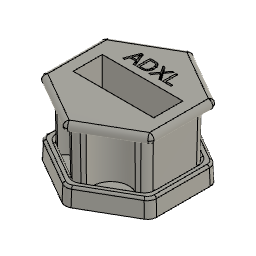
EXPAND CONNECTER v5 (Autodesk Fusion 360 design; units mm, degrees)
Autodesk Fusion 360 part; units mm, degrees
sketch "草图1" plane through (0, 0, 0) normal (0, 0, 1) x (1, 0, 0)
  line L0 (10.3777, -5.9969) -> (10.3823, 5.9889)
  line L1 (10.3823, 5.9889) -> (0.0046, 11.9858)
  line L2 (0.0046, 11.9858) -> (-10.3777, 5.9969)
  line L3 (-10.3777, 5.9969) -> (-10.3823, -5.9889)
  line L4 (-10.3823, -5.9889) -> (-0.0046, -11.9858)
  line L5 (-0.0046, -11.9858) -> (10.3777, -5.9969)
  line L6 (9, -3.25) -> (-9, -3.25)
  line L7 (-9, -3.25) -> (-9, 3.25)
  line L8 (-9, 3.25) -> (9, 3.25)
  line L9 (9, 3.25) -> (9, -3.25)
  line L10 (9, -3.25) -> (-9, 3.25) construction
  line L11 (-9, -3.25) -> (9, 3.25) construction
  line L12 (8, 2.925) -> (-8, 2.925) construction
  line L13 (-8, 3.25) -> (-8, -2.925) construction
  line L14 (-8, -2.925) -> (8, -2.925) construction
  line L15 (8, -2.925) -> (8, 3.25) construction
  line L16 (8, 2.925) -> (-8, -2.925) construction
  line L17 (-8, 2.925) -> (8, -2.925) construction
  line L18 (8, 3.25) -> (-8, 3.25)
  line L19 (-8, 3.25) -> (-8, -2.6)
  line L20 (-8, -2.6) -> (8, -2.6)
  line L21 (8, -2.6) -> (8, 3.25)
  line L22 (-12.3772, 7.1524) -> (-12.3828, -7.1428)
  line L23 (-12.3828, -7.1428) -> (-0.0055, -14.2952)
  line L24 (-0.0055, -14.2952) -> (12.3772, -7.1524)
  line L25 (12.3772, -7.1524) -> (12.3828, 7.1428)
  line L26 (12.3828, 7.1428) -> (0.0055, 14.2952)
  line L27 (0.0055, 14.2952) -> (-12.3772, 7.1524)
  circle A0 centre (-5.1935, -8.9873) radius 4
  circle A1 centre (5.1865, -8.9914) radius 4
  circle A2 centre (-5.1865, 8.9914) radius 4
  circle A3 centre (5.1935, 8.9873) radius 4
  line L28 (-5.1935, -8.9873) -> (-1.8781, -3.25) construction
  line L29 (5.1865, -8.9914) -> (1.8747, -3.25) construction
  point P0 (-3.5358, -6.1187)
  point P1 (3.5306, -6.1207)
  dimension "d5" = 10.38
  dimension "d6" = 18
  dimension "d7" = 6.5
  dimension "d8" = 16
  dimension "d9" = 5.85
  dimension "d10" = 5.85
  dimension "d11" = 2
  dimension "d28" = 8
  dimension "d29" = 8
  dimension "d30" = 8
  dimension "d31" = 8
  constraint horizontal L6
  constraint perpendicular L6 L7
  constraint parallel L6 L8
  constraint parallel L7 L9
  constraint coincident L10 origin
  constraint coincident L11 origin
  constraint horizontal L12
  constraint perpendicular L12 L13
  constraint parallel L12 L14
  constraint parallel L13 L15
  constraint coincident L16 origin
  constraint coincident L17 origin
  constraint coincident L12.end L13
  constraint coincident L8 L13.start
  constraint coincident L12.start L15
  constraint coincident L8 L15.end
  constraint horizontal L18
  constraint vertical L19
  constraint horizontal L20
  constraint vertical L21
  constraint midpoint L4 A0.centre
  constraint midpoint L5 A1.centre
  constraint midpoint L2 A2.centre
  constraint midpoint L1 A3.centre
  constraint coincident A0.centre L28.start
  constraint coincident L6 L28.end
  constraint perpendicular L4 L28
  constraint coincident A1.centre L29.start
  constraint coincident L6 L29.end
  constraint perpendicular L5 L29
  constraint midpoint L28 P0
  constraint midpoint L29 P1
  measures "d5" distance of origin L5
  measures "d6" distance of L7.end L8.end
  measures "d7" distance of L6.end L7.end
  measures "d8" distance of L13.end L14.end
  measures "d9" distance of L12.end L13.end
  measures "d10" distance of L15.end L20.end
  measures "d28" diameter of A0
  measures "d29" diameter of A1
  measures "d30" diameter of A2
  measures "d31" diameter of A3
extrude "拉伸1" add sketch "草图1" along normal blind 14.2 draft 1 contours L0 L1 L2 L3 L4 L5 A0 A1 A2 A3 | L5 A1 | L1 A3 | L4 A0 | L2 A2 | L6 L7 L8 L9 L19 L20 L21 | L8 L18 L19 L20 L21 makes body 1
extrude "拉伸2" add sketch "草图1" along normal blind 2 from surface at 14.2 contours L0 L1 L2 L3 L4 L5 A0 A1 A2 A3 | L0 L1 L5 L24 L25 L26 A1 A3 | L5 L24 A1 | L5 A1 | L1 A3 | L1 L26 A3 | L4 L5 L23 L24 A0 A1 | L1 L2 L26 L27 A2 A3 | L4 L23 A0 | L4 A0 | L2 A2 | L2 L27 A2 | L2 L3 L4 L22 L23 L27 A0 A2 bodies 1
extrude "拉伸3" cut sketch "草图1" along normal blind 7.8 contours L8 L18 L19 L20 L21 bodies 1
extrude "拉伸4" cut sketch "草图1" along normal blind 12 from surface at 7.8 contours L6 L7 L8 L9 L19 L20 L21 | L8 L18 L19 L20 L21 bodies 1
fillet "圆角1" radius 2 1 edges at (-0.0047, -12.1289, 7.1) on bodies 1
fillet "圆角2" radius 2 5 edges at (10.5063, 6.0604, 7.1) (10.5016, -6.0685, 7.1) (0.0047, 12.1289, 7.1) (-10.5016, 6.0685, 7.1) (-10.5063, -6.0604, 7.1) on bodies 1
fillet "圆角3" radius 1 18 edges at (-0.0055, -14.2952, 15.2) (12.3772, -7.1524, 15.2) (12.3828, 7.1428, 15.2) (0.0055, 14.2952, 15.2) (-12.3772, 7.1524, 15.2) (-12.3828, -7.1428, 15.2) (-6.1941, -10.719, 16.2) (-6.1941, -10.719, 14.2) (6.1859, -10.7238, 14.2) (6.1859, -10.7238, 16.2) (-12.38, 0.0048, 14.2) (-12.38, 0.0048, 16.2) (12.38, -0.0048, 16.2) (12.38, -0.0048, 14.2) (6.1941, 10.719, 16.2) (6.1941, 10.719, 14.2) (-6.1859, 10.7238, 16.2) (-6.1859, 10.7238, 14.2) on bodies 1
extrude "拉伸5" cut sketch "草图1" along normal blind 12 from surface at 2 contours L5 L24 A1 | L5 A1 | L1 A3 | L1 L26 A3 | L4 L23 A0 | L4 A0 | L2 A2 | L2 L27 A2 bodies 1
sketch "草图2" plane through (0, 0, 0) normal (0, 0, 1) x (1, 0, 0)
  line L0 (-6.0005, 4.5625) -> (7.0007, 4.5463) construction
  line L1 (7.0007, 4.5463) -> (7.0048, 7.8088) construction
  line L2 (7.0048, 7.8088) -> (-5.9964, 7.8251) construction
  line L3 (-5.9964, 7.8251) -> (-6.0005, 4.5625) construction
  point P0 (-5.9964, 7.8251)
  dimension "d40" = 3
  text T0 "ADXL" font "Arial" height 3 align left top in box 13.0012 x 3.2625 at (-6.0005, 4.5625) x (0.999999, -0.001251) y (0.001251, 0.999999) spacing 1
  constraint coincident P0
extrude "拉伸7" cut sketch "草图2" against normal blind 1 from surface at 16.2 text T0 bodies 1
sketch "草图3" plane through (0, 0, 0) normal (0, 0, 1) x (1, 0, 0)
  line L0 (-5.9964, 4.5463) -> (7.0007, 4.5463) construction
  line L1 (7.0007, 4.5463) -> (7.0007, 7.8251) construction
  line L2 (7.0007, 7.8251) -> (-5.9964, 7.8251) construction
  line L3 (-5.9964, 7.8251) -> (-5.9964, 4.5463) construction
  point P0 (-5.9964, 7.8251)
  point P1 (7.0007, 4.5463)
  dimension "d44" = 3
  constraint coincident P1
  constraint coincident P0
extrude "拉伸8" [suppressed]
extrude "拉伸9" add sketch "草图1" along normal blind 4 draft -2 separate body contours L0 L1 L5 L24 L25 L26 A1 A3 | L5 L24 A1 | L1 L26 A3 | L4 L5 L23 L24 A0 A1 | L1 L2 L26 L27 A2 A3 | L4 L23 A0 | L2 L27 A2 | L2 L3 L4 L22 L23 L27 A0 A2 makes body 2
fillet "圆角4" radius 2 12 edges at (-10.4475, 6.0373, 2) (-10.4522, -6.0292, 2) (-0.0047, -12.0664, 2) (10.4475, -6.0373, 2) (10.4522, 6.0292, 2) (0.0047, 12.0664, 2) (-12.3074, 7.112, 2) (0.0055, 14.2145, 2) (-12.3129, -7.1025, 2) (-0.0055, -14.2145, 2) (12.3074, -7.112, 2) (12.3129, 7.1025, 2) on bodies 2
fillet "圆角5" radius 0.5 24 edges at (12.2403, -0.0047, 4) (11.9699, -6.917, 4) (6.1161, -10.6028, 4) (-0.0053, -13.8247, 4) (-6.1243, -10.5981, 4) (-11.9752, -6.9077, 4) (-12.2403, 0.0047, 4) (-11.9699, 6.917, 4) (-6.1161, 10.6028, 4) (0.0053, 13.8247, 4) (6.1243, 10.5981, 4) (11.9752, 6.9077, 4) (10.2496, -5.9229, 4) (5.2563, -9.1123, 4) (-0.0046, -11.8379, 4) (-5.2634, -9.1083, 4) (-10.2542, -5.915, 4) (-10.5197, 0.0041, 4) (-10.2496, 5.9229, 4) (-5.2563, 9.1123, 4) (0.0046, 11.8379, 4) (5.2634, 9.1083, 4) (10.2542, 5.915, 4) (10.5197, -0.0041, 4) on bodies 2
